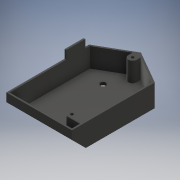
# Autodesk Inventor part: AC03
Saved by Autodesk Inventor 2017 (Build 210142000, 142)
## iProperties
Created: 2019-08-28
Part Number: AC03
Material: ABS Plastic
Document SubType Name: Modeling
Designer: Dell
Density: 1.06 g/cm^3
Appearance: Smooth - Black
Author: Dell
Autodesk Inventor part; units mm, degrees
ref_plane "YZ Plane" through (0, 0, 0) normal (1, 0, 0) x (0, 1, 0)
ref_plane "XZ Plane" through (0, 0, 0) normal (0, 1, 0) x (-1, 0, 0)
ref_plane "XY Plane" through (0, 0, 0) normal (0, 0, 1) x (1, 0, 0)
sketch "Sketch1" plane through (0, 0, 0) normal (0, 0, 1) x (1, 0, 0)
  line L0 (0, 68.1273) -> (59, 34.0637)
  line L1 (59, 34.0637) -> (59, -34.0637)
  line L2 (59, -34.0637) -> (0, -68.1273)
  line L3 (0, -68.1273) -> (-59, -34.0637)
  line L4 (-59, -34.0637) -> (-59, 34.0637)
  line L5 (-59, 34.0637) -> (0, 68.1273)
  line L6 (-59, -34.0637) -> (-59, -115)
  line L7 (-59, -115) -> (59, -115)
  line L8 (59, -115) -> (59, -34.0637)
  point P0 (0, 0)
  point P1 (0, 0)
  dimension "d0" = 118
  dimension "d1" = 115
  constraints: 18 end point, 2 perpendicular, 1 coincident, 1 vertical, 1 vertical alignment, 13 other
  measures "d0" distance between parallel lines of L1 L4
  measures "d1" distance from line of L7 point (0, 0)
extrude "Extrusion1" add sketch "Sketch1" along normal blind 5
sketch "Sketch2" plane through (0, 0, 5) normal (0, 0, 1) x (1, 0, 0)
  line L0 (59, -115) -> (59, 34.0637) projected
  line L1 (59, 34.0637) -> (0, 68.1273) projected
  line L2 (0, 68.1273) -> (-59, 34.0637) projected
  line L3 (-59, 34.0637) -> (-59, -115) projected
  line L4 (-59, -115) -> (59, -115) projected
  line L5 (-56, 32.3316) -> (0, 64.6632)
  line L6 (0, 64.6632) -> (56, 32.3316)
  line L7 (56, 32.3316) -> (56, -112)
  line L8 (56, -112) -> (-56, -112)
  line L9 (-56, -112) -> (-56, 32.3316)
  point P0 (0, 0)
  dimension "d4" = 3
  constraints: 10 end point, 4 other
  measures "d4" distance between parallel lines of L2 L5
extrude "Extrusion2" add sketch "Sketch2" along normal blind 35
sketch "Sketch3" plane through (0, 0, 0) normal (0, 0, -1) x (-1, 0, 0)
  circle A0 centre (0, 53.1273) radius 2.5
  circle A1 centre (-34, -90) radius 2.5
  line L0 (59, -115) -> (-59, -115) projected
  line L1 (-59, -115) -> (-59, 34.0637) projected
  point P0 (0, 0)
  point P1 (0, 68.1273)
  dimension "d7" = 5
  dimension "d8" = 5
  dimension "d9" = 25
  dimension "d10" = 25
  dimension "d11" = 15
  constraints: 2 centre point, 1 vertical alignment
  measures "d7" diameter of A0
  measures "d8" diameter of A1
  measures "d9" distance from line of L0 A1.centre
  measures "d10" distance from line of A1.centre L1
  measures "d11" distance of A0.centre point (0, 68.127)
extrude "Extrusion3" cut sketch "Sketch3" against normal through all
sketch "Sketch5" plane through (0, 0, 5) normal (0, 0, 1) x (1, 0, 0)
  circle A0 centre (0, 53.1273) radius 2.5 projected
  circle A1 centre (0, 53.1273) radius 7.5
  circle A2 centre (34, -90) radius 2.5 projected
  circle A3 centre (34, -90) radius 7.5
  point P0 (0, 0)
  dimension "d19" = 15
  dimension "d20" = 15
  constraints: 2 centre point, 2 coincident
  measures "d19" diameter of A1
  measures "d20" diameter of A3
extrude "Extrusion5" add sketch "Sketch5" along normal up to surface (35 mm away) from surface at 0
sketch "Sketch6" plane through (0, 0, 0) normal (0, 0, -1) x (-1, 0, 0)
  circle A0 centre (0, 0) radius 7.5
  circle A1 centre (-19.799, -19.799) radius 4
  circle A2 centre (-21.2132, 21.2132) radius 4
  circle A3 centre (19.799, 19.799) radius 5
  line L0 (0, 0) -> (32.276, 0) construction
  line L1 (0, 0) -> (-19.799, -19.799) construction
  line L2 (0, 0) -> (-21.2132, 21.2132) construction
  line L3 (0, 0) -> (19.799, 19.799) construction
  line L4 (10.799, 27.799) -> (28.799, 27.799) construction
  line L5 (28.799, 27.799) -> (28.799, -5.201) construction
  line L6 (28.799, -5.201) -> (10.799, -5.201) construction
  line L7 (10.799, -5.201) -> (10.799, 27.799) construction
  circle A4 centre (10.799, 27.799) radius 1.75
  circle A5 centre (28.799, 27.799) radius 1.75
  circle A6 centre (28.799, -5.201) radius 1.75
  circle A7 centre (10.799, -5.201) radius 1.75
  point P0 (19.799, 27.799)
  dimension "d23" = 15
  dimension "d24" = 8
  dimension "d25" = 8
  dimension "d26" = 10
  dimension "d27" = 28
  dimension "d28" = 30
  dimension "d29" = 28
  dimension "d30" = 45
  dimension "d31" = 18
  dimension "d32" = 33
  dimension "d33" = 8
  dimension "d34" = 3.5
  dimension "d35" = 3.5
  dimension "d36" = 3.5
  dimension "d37" = 3.5
  dimension "d38" = 135
  dimension "d39" = 135
  constraints: 16 end point, 8 centre point, 6 coincident, 2 horizontal, 2 parallel, 1 midpoint, 1 perpendicular, 1 vertical alignment
  measures "d23" diameter of A0
  measures "d24" diameter of A1
  measures "d25" diameter of A2
  measures "d26" diameter of A3
  measures "d27" distance of point (0, 0) L3.end
  measures "d28" distance of point (0, 0) L2.end
  measures "d29" distance of point (0, 0) L1.end
  measures "d30" angle of L0 L3
  measures "d31" distance of L4.start L4.end
  measures "d32" distance of L4.end L5.end
  measures "d33" distance from line of L4 L3.end
  measures "d34" diameter of A4
  measures "d35" diameter of A5
  measures "d36" diameter of A6
  measures "d37" diameter of A7
  measures "d38" angle of L0 L1
  measures "d39" angle of L2 L0
extrude "Extrusion6" cut sketch "Sketch6" against normal through all contours A3
sketch "Sketch8" plane through (0, 0, 40) normal (0, 0, 1) x (1, 0, 0)
  line L0 (-56, -112) -> (-56, 32.3316) projected
  line L1 (-59, 24.0637) -> (-56, 24.0637)
  line L2 (-56, 24.0637) -> (-56, -9.9363)
  line L3 (-56, -9.9363) -> (-59, -9.9363)
  line L4 (-59, -9.9363) -> (-59, 24.0637)
  line L5 (-59, 34.0637) -> (-59, -115) projected
  point P0 (0, 0)
  dimension "d42" = 10
  dimension "d43" = 34
  constraints: 8 end point, 2 parallel, 2 point on line, 1 horizontal, 1 perpendicular
  measures "d42" distance from line of L5.start L1
  measures "d43" distance between parallel lines of L1 L3
extrude "Extrusion7" add sketch "Sketch8" along normal blind 15
chamfer "Chamfer1" distance 25 angle 45 1 edges at (0, -115, 0)
sketch "Sketch9" plane through (59, -115, 25) normal (0, -0.7071068, -0.7071068) x (-1, 0, 0)
  line L0 (3, 4.2426) -> (3, 28.2843) projected
  line L1 (3, 28.2843) -> (19.4098, 28.2843) projected
  ellipse E0 centre (25, 35.3553) end of major axis (25, 24.7487) minor radius 7.5 (19.4098, 28.2843) -> (30.5902, 28.2843) ccw projected
  line L2 (30.5902, 28.2843) -> (115, 28.2843) projected
  line L3 (115, 28.2843) -> (115, 4.2426) projected
  line L4 (115, 4.2426) -> (3, 4.2426) projected
  line L5 (0, 35.3553) -> (0, 0) projected
  line L6 (0, 0) -> (118, 0) projected
  line L7 (118, 0) -> (118, 35.3553) projected
  line L8 (118, 35.3553) -> (27.5, 35.3553) projected
  ellipse E1 centre (25, 35.3553) end of major axis (25, 38.8909) minor radius 2.5 (22.5, 35.3553) -> (27.5, 35.3553) ccw projected
  line L9 (22.5, 35.3553) -> (0, 35.3553) projected
  point P0 (59, 98.9949)
  constraints: 2 other
extrude "Extrusion8" add sketch "Sketch9" against normal blind 3 contours L0 L1 E0 L2 L3 L4 | L9 E1 L8 L7 L6 L5
sketch "Sketch10" plane through (0, 0, 0) normal (0, 0, -1) x (-1, 0, 0)
  arc A0 (-31.5, -90) -> (-36.5, -90) centre (-34, -90) ccw projected
  circle A1 centre (-34, -90) radius 2.5
  point P0 (0, 0)
  constraints: 1 coincident, 1 horizontal alignment, 2 other
extrude "Extrusion9" cut sketch "Sketch10" against normal through all
sketch "Sketch12" plane through (0, 0, 0) normal (0, 0, -1) x (-1, 0, 0)
  arc A0 (-31.5, -90) -> (-36.5, -90) centre (-34, -90) ccw projected
  circle A1 centre (-34, -90) radius 2.5
  circle A2 centre (-34, -90) radius 2.5 projected
  circle A3 centre (-34, -90) radius 6.5
  point P0 (0, 0)
  dimension "d53" = 13
  constraints: 2 coincident, 1 centre point, 1 horizontal alignment, 2 other
  measures "d53" diameter of A3
extrude "Extrusion10" cut sketch "Sketch12" against normal blind 10
sketch "Sketch13" plane through (0, 0, 0) normal (0, 0, -1) x (-1, 0, 0)
  circle A0 centre (0, 53.1273) radius 2.5 projected
  circle A1 centre (0, 53.1273) radius 6.5
  point P0 (0, 0)
  dimension "d56" = 13
  constraints: 1 centre point, 1 coincident
  measures "d56" diameter of A1
extrude "Extrusion11" cut sketch "Sketch13" against normal blind 10
sketch "Sketch15" plane through (0, 0, 5) normal (0, 0, 1) x (1, 0, 0)
  circle A0 centre (0, 53.1273) radius 7.5 projected
  line L0 (-56, 32.3316) -> (0, 64.6632) projected
  line L1 (0, 64.6632) -> (56, 32.3316) projected
  line L2 (-7.5, 53.1273) -> (-7.5, 60.3331)
  line L3 (-7.5, 60.3331) -> (0, 64.6632)
  line L4 (0, 64.6632) -> (7.5, 60.3331)
  line L5 (7.5, 53.1273) -> (7.5, 60.3331)
  arc A1 (7.5, 53.1273) -> (-7.5, 53.1273) centre (0, 53.1273) ccw
  point P0 (0, 0)
  constraints: 8 end point, 4 point on circle, 4 tangent, 2 point on line, 1 centre point, 1 parallel, 1 vertical
extrude "Extrusion12" add sketch "Sketch15" along normal up to surface (35 mm away) from surface at 0 contours A0 L2 L0 L1 L5
sketch "Sketch16" plane through (0, 0, 5) normal (0, 0, 1) x (1, 0, 0)
  circle A0 centre (34, -90) radius 7.5 projected
  circle A1 centre (34, -90) radius 2.5 projected
  line L0 (34, -82.5) -> (59, -82.5)
  line L1 (59, -90) -> (59, 34.0637) projected
  line L2 (59, -82.5) -> (59, -97.5)
  line L3 (59, -97.5) -> (34, -97.5)
  arc A2 (34, -97.5) -> (34, -82.5) centre (34, -90) ccw
  point P0 (0, 0)
  constraints: 6 end point, 4 point on circle, 4 tangent, 2 horizontal, 1 centre point, 1 point on line, 1 vertical
extrude "Extrusion13" add sketch "Sketch16" along normal up to surface (35 mm away) from surface at 0 contours A0 L0 L1 L2 L3
sketch "Sketch17" plane through (-59, 34.0637, 0) normal (-1, 0, 0) x (0, 0, 1)
  line L0 (5, -129.0637) -> (7.5, -131.5637) projected
  line L1 (5, -131.5637) -> (5, -129.0637) projected
  line L2 (5, -131.5637) -> (7.5, -131.5637) projected
  point P0 (0, -34.0637)
extrude "Extrusion14" cut sketch "Sketch17" against normal through all
equation "\"d34\" = d36"
equation "\"d35\" = d36"
equation "\"d37\" = d36"
body "Solid1"
